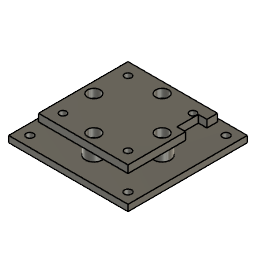
FC_TRAY (Autodesk Fusion 360 design; units mm, degrees)
Autodesk Fusion 360 part; units mm, degrees
note: some values were not read from the file. Chosen so that the rebuilt part matches the saved one: which bodies a step acts on.
sketch "Sketch1" plane through (0, 0, 0) normal (0, 0, 1) x (1, 0, 0) in component "FC_TRAY_V1"
  line L0 (-28, -28) -> (28, -28)
  line L1 (28, -28) -> (28, 28)
  line L2 (28, 28) -> (-28, 28)
  line L3 (-28, 28) -> (-28, -28)
extrude "Extrude1" add sketch "Sketch1" along normal blind 3 makes body 1 in component "FC_TRAY_V1"
sketch "Sketch2" plane through (0, 0, 0) normal (0, 0, 1) x (1, 0, 0) in component "FC_TRAY_V1"
  circle A0 centre (16, 0) radius 4
  circle A1 centre (-16, 0) radius 4
  circle A2 centre (0, 16) radius 4
  circle A3 centre (0, -16) radius 4
extrude "Extrude2" add sketch "Sketch2" along normal blind 6.5 from surface at 2.5 separate body makes body 2 at (3.9801, 15.6017, 6.8333) makes body 3 at (-12.0199, -0.3983, 6.8333) makes body 4 at (19.9801, -0.3983, 6.8333) makes body 5 at (3.9801, -16.3983, 6.8333) in component "FC_TRAY_V1"
sketch "Sketch3" plane through (0, 0, 0) normal (0, 0, 1) x (1, 0, 0) in component "FC_TRAY_V1"
  line L0 (-21, -21) -> (21, -21)
  line L1 (21, -21) -> (21, 21)
  line L2 (21, 21) -> (-21, 21)
  line L3 (-21, 21) -> (-21, -21)
extrude "Extrude3" add sketch "Sketch3" along normal blind 3.5 from surface at 8.5 separate body makes body 6 in component "FC_TRAY_V1"
combine "Combine1" operation add target body 1 tool bodies 2 3 4 5 6 in component "FC_TRAY_V1"
sketch "Sketch4" plane through (0, 0, 0) normal (0, 0, 1) x (1, 0, 0) in component "FC_TRAY_V1"
  circle A0 centre (23, 23) radius 1.7
  circle A1 centre (-23, 23) radius 1.7
  circle A2 centre (23, -23) radius 1.7
  circle A3 centre (-23, -23) radius 1.7
extrude "Extrude4" cut sketch "Sketch4" along normal blind 5 from surface at -1 bodies 1 in component "FC_TRAY_V1"
sketch "Sketch5" plane through (0, 0, 0) normal (0, 0, 1) x (1, 0, 0) in component "FC_TRAY_V1"
  circle A0 centre (15.25, 15.25) radius 1.6
  circle A1 centre (-15.25, 15.25) radius 1.6
  circle A2 centre (15.25, -15.25) radius 1.6
  circle A3 centre (-15.25, -15.25) radius 1.6
extrude "Extrude5" cut sketch "Sketch5" along normal blind 5 from surface at 8 bodies 1 in component "FC_TRAY_V1"
sketch "Sketch6" plane through (0, 0, 0) normal (0, 0, 1) x (1, 0, 0) in component "FC_TRAY_V1"
  circle A0 centre (16, 0) radius 3
  circle A1 centre (-16, 0) radius 3
  circle A2 centre (0, 16) radius 3
  circle A3 centre (0, -16) radius 3
extrude "Extrude6" cut sketch "Sketch6" along normal blind 4 from surface at 8 bodies 1 in component "FC_TRAY_V1"
sketch "Sketch7" plane through (0, 0, 0) normal (0, 0, 1) x (1, 0, 0) in component "FC_TRAY_V1"
  line L0 (17, 6) -> (21, 6)
  line L1 (21, 6) -> (21, 16)
  line L2 (21, 16) -> (17, 16)
  line L3 (17, 16) -> (17, 6)
extrude "Extrude7" cut sketch "Sketch7" along normal blind 5 from surface at 8 bodies 1 in component "FC_TRAY_V1"
component "FC_TRAY_V1" placed x (1, 0, 0) y (0, 1, 0) z (0, 0, 1) at (0, 0, 0)
